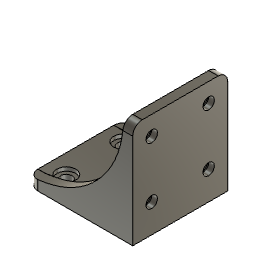
_body bracket v1.9dabf268-07d1-46ed-89ed-1b83d9925f87 (Autodesk Fusion 360 design; units mm, degrees)
Autodesk Fusion 360 part; units mm, degrees
note: some values were not read from the file. Set by a fixed rule: which sketch regions a step uses.
sketch "Sketch1" plane through (0, 0, 0) normal (0, 0, 1) x (1, 0, 0)
  line L0 (0, 0) -> (55, 0)
  line L1 (55, 0) -> (55, 50)
  line L2 (55, 50) -> (0, 50)
  line L3 (0, 50) -> (0, 0)
  dimension "d1" = 55
  dimension "d2" = 50
  constraint horizontal L0
  constraint vertical L1
  constraint horizontal L2
  constraint vertical L3
  constraint coincident L0.start L3.end
  measures "d1" distance of L0.start L0.end
  measures "d2" distance of L0.start L2.end
extrude "Extrude1" add sketch "Sketch1" along normal blind 5
sketch "Sketch2" plane through (0, 0, 5) normal (0, 0, 1) x (-1, 0, 0)
  line L0 (0, -50) -> (0, 0)
  line L1 (0, 0) -> (-55, 0)
  line L2 (-55, 0) -> (-55, -50)
  line L3 (-55, -50) -> (0, -50)
  circle A0 centre (-10, -40) radius 3
  circle A1 centre (-10, -10) radius 3
  circle A2 centre (-40, -10) radius 3
  circle A3 centre (-40, -40) radius 3
  dimension "d5" = 6
  dimension "d6" = 6
  dimension "d7" = 6
  dimension "d8" = 6
  measures "d5" diameter of A0
  measures "d6" diameter of A1
  measures "d7" diameter of A2
  measures "d8" diameter of A3
extrude "Extrude2" cut sketch "Sketch2" against normal blind 5 contours A0 | A1 | A2 | A3
sketch "Sketch3" plane through (0, 0, 5) normal (0, 0, 1) x (-1, 0, 0)
  circle A0 centre (-40, -40) radius 3
  circle A1 centre (-40, -10) radius 3
  circle A2 centre (-10, -40) radius 3
  circle A3 centre (-10, -10) radius 3
  line L0 (0, -50) -> (0, 0)
  line L1 (0, 0) -> (-55, 0)
  line L2 (-55, 0) -> (-55, -50)
  line L3 (-55, -50) -> (0, -50)
  circle A4 centre (-10, -10) radius 5
  circle A5 centre (-10, -40) radius 5
  circle A6 centre (-40, -40) radius 5
  circle A7 centre (-40, -10) radius 5
  dimension "d11" = 10
  dimension "d12" = 10
  dimension "d13" = 10
  dimension "d14" = 10
  constraint concentric A3 A4
  constraint concentric A2 A5
  constraint concentric A0 A6
  constraint concentric A1 A7
  measures "d11" diameter of A4
  measures "d12" diameter of A5
  measures "d13" diameter of A6
  measures "d14" diameter of A7
extrude "Extrude3" cut sketch "Sketch3" against normal blind 2 contours A4 | A5 | A6 | A7
sketch "Sketch4" plane through (0, 0, 5) normal (0, 0, 1) x (-1, 0, 0)
  circle A0 centre (-40, -40) radius 5
  circle A1 centre (-40, -10) radius 5
  circle A2 centre (-10, -40) radius 5
  circle A3 centre (-10, -10) radius 5
  line L0 (0, -50) -> (0, 0)
  line L1 (0, 0) -> (-55, 0)
  line L2 (-55, 0) -> (-55, -50)
  line L3 (-55, -50) -> (0, -50)
  line L4 (-50, 0) -> (-55, 0)
  line L5 (-55, 0) -> (-55, -50)
  line L6 (-55, -50) -> (-50, -50)
  line L7 (-50, -50) -> (-50, 0)
  dimension "d17" = 5
  dimension "d18" = 50
  constraint horizontal L4
  constraint vertical L5
  constraint horizontal L6
  constraint vertical L7
  constraint coincident L1 L4.start
  measures "d17" distance of L4.start L1.end
  measures "d18" distance of L4.start L6.end
extrude "Extrude4" add sketch "Sketch4" along normal blind 50 contours L1 L2 L3 L4 L5 L6 L7
sketch "Sketch5" plane through (50, 0, 0) normal (-1, 0, 0) x (0, -1, 0)
  line L0 (-50, 5) -> (0, 5)
  line L1 (0, 5) -> (0, 55)
  line L2 (0, 55) -> (-50, 55)
  line L3 (-50, 55) -> (-50, 5)
  circle A0 centre (-40, 45) radius 3
  circle A1 centre (-10, 45) radius 3
  circle A2 centre (-10, 15) radius 3
  circle A3 centre (-40, 15) radius 3
  dimension "d21" = 6
  dimension "d22" = 6
  dimension "d23" = 6
  dimension "d24" = 6
  measures "d21" diameter of A0
  measures "d22" diameter of A1
  measures "d23" diameter of A2
  measures "d24" diameter of A3
extrude "Extrude5" cut sketch "Sketch5" against normal blind 5 contours A0 | A1 | A2 | A3
sketch "Sketch6" plane through (50, 0, 0) normal (-1, 0, 0) x (0, -1, 0)
  circle A0 centre (-10, 45) radius 3
  circle A1 centre (-10, 15) radius 3
  circle A2 centre (-40, 45) radius 3
  circle A3 centre (-40, 15) radius 3
  line L0 (-50, 5) -> (0, 5)
  line L1 (0, 5) -> (0, 55)
  line L2 (0, 55) -> (-50, 55)
  line L3 (-50, 55) -> (-50, 5)
  circle A4 centre (-40, 45) radius 5
  circle A5 centre (-10, 45) radius 5
  circle A6 centre (-40, 15) radius 5
  circle A7 centre (-10, 15) radius 5
  dimension "d27" = 10
  dimension "d28" = 10
  dimension "d29" = 10
  dimension "d30" = 10
  constraint concentric A2 A4
  constraint concentric A0 A5
  constraint concentric A3 A6
  constraint concentric A1 A7
  measures "d27" diameter of A4
  measures "d28" diameter of A5
  measures "d29" diameter of A6
  measures "d30" diameter of A7
extrude "Extrude6" cut sketch "Sketch6" against normal blind 2 contours A4 | A5 | A6 | A7
sketch "Sketch7" plane through (0, 0, 0) normal (0, -1, 0) x (1, 0, 0)
  line L0 (0, 0) -> (55, 0)
  line L1 (55, 0) -> (55, 55)
  line L2 (55, 55) -> (50, 55)
  line L3 (50, 55) -> (50, 5)
  line L4 (50, 5) -> (0, 5)
  line L5 (0, 5) -> (0, 0)
  line L6 (55, 0) -> (0, 0)
  line L7 (0, 0) -> (0, 55)
  line L8 (0, 55) -> (55, 55)
  line L9 (55, 55) -> (55, 0)
  constraint horizontal L6
  constraint vertical L7
  constraint horizontal L8
  constraint vertical L9
  constraint coincident L0.end L1.start
extrude "Extrude7" add sketch "Sketch7" against normal blind 5 contours L3 L4 L7 L8
sketch "Sketch8" plane through (0, 50, 0) normal (0, 1, 0) x (-1, 0, 0)
  line L0 (-55, 0) -> (0, 0)
  line L1 (0, 0) -> (0, 5)
  line L2 (0, 5) -> (-50, 5)
  line L3 (-50, 5) -> (-50, 55)
  line L4 (-50, 55) -> (-55, 55)
  line L5 (-55, 55) -> (-55, 0)
  line L6 (0, 55) -> (-55, 55)
  line L7 (-55, 55) -> (-55, 0)
  line L8 (-55, 0) -> (0, 0)
  line L9 (0, 0) -> (0, 55)
  constraint horizontal L6
  constraint vertical L7
  constraint horizontal L8
  constraint vertical L9
  constraint coincident L0.start L5.end
extrude "Extrude8" add sketch "Sketch8" against normal blind 5 contours L2 L3 L6 L9
sketch "Sketch9" plane through (0, 50, 0) normal (0, 1, 0) x (-1, 0, 0)
  line L0 (-55, 0) -> (0, 0)
  line L1 (0, 0) -> (0, 55)
  line L2 (0, 55) -> (-55, 55)
  line L3 (-55, 55) -> (-55, 0)
  circle A0 centre (0, 55) radius 50
  constraint coincident L1.end L2.start
extrude "Extrude9" cut sketch "Sketch9" against normal blind 50 contours L1 L2 A0 | L1 L2 A0
fillet "Fillet1" radius 5 4 edges at (0, 0, 2.5) (52.5, 0, 55) (52.5, 50, 55) (0, 50, 2.5)
